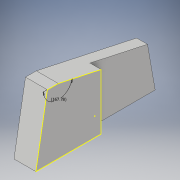
# Autodesk Inventor part: SideProfile
Saved by Autodesk Inventor 2019 (Build 230136000, 136)
## iProperties
Created: 2019-01-04
Part Number: SideProfile
Material: Generic
Document SubType Name: Modeling
Designer: james
Density: 1 g/cm^3
Appearance: Default
Author: james
Autodesk Inventor part; units mm, degrees
ref_plane "YZ Plane" through (0, 0, 0) normal (1, 0, 0) x (0, 1, 0)
ref_plane "XZ Plane" through (0, 0, 0) normal (0, 1, 0) x (-1, 0, 0)
ref_plane "XY Plane" through (0, 0, 0) normal (0, 0, 1) x (1, 0, 0)
sketch "Sketch1" plane through (0, 0, 0) normal (1, 0, 0) x (0, 1, 0)
  line L0 (-43.7628, 137.6658) -> (-43.7628, -167.1342)
  line L1 (-43.7628, -167.1342) -> (57.8372, -149.2194)
  line L2 (-43.7628, 137.6658) -> (108.6372, 110.7936)
  line L3 (108.6372, 110.7936) -> (108.6372, 85.3936)
  line L4 (108.6372, 85.3936) -> (57.8372, -149.2194)
  point P0 (0, 0)
  dimension "d0" = 80
  dimension "d1" = 304.8
  dimension "d2" = 101.6
  dimension "d3" = 80
  dimension "d4" = 152.4
  dimension "d5" = 25.4
  constraints: 10 end point, 2 vertical
  measures "d0" angle of L0 L1
  measures "d1" distance of L0.start L0.end
  measures "d2" distance from line of L0 L1.end
  measures "d3" angle of L2 L0
  measures "d4" distance from line of L0 L2.end
  measures "d5" distance of L2.end L3.end
extrude "Extrusion1" add sketch "Sketch1" along normal blind 25.4
sketch "Sketch2" plane through (25.4, 0, 0) normal (1, 0, 0) x (0, 0, -1)
  line L0 (-137.6658, -43.7628) -> (14.7342, -43.7628)
  line L1 (-137.6658, -43.7628) -> (167.1342, -43.7628) projected
  line L2 (14.7342, -43.7628) -> (14.7342, 86.9569)
  line L3 (149.2194, 57.8372) -> (-85.3936, 108.6372) projected
  line L4 (-85.3936, 108.6372) -> (-110.7936, 108.6372) projected
  line L5 (-110.7936, 108.6372) -> (-137.6658, -43.7628) projected
  point P0 (0, 0)
  dimension "d8" = 152.4
  dimension "d9" = 0
  constraints: 4 end point, 1 midpoint, 1 point on line, 1 vertical
  measures "d8" distance of L0.start L0.end
  measures "d9" distance of L1.start L0.start
extrude "Extrusion2" add sketch "Sketch2" along normal blind 25.4
sketch "Sketch3" plane through (50.8, 0, 0) normal (1, 0, 0) x (0, 0, -1)
  line L0 (-85.3936, 108.6372) -> (-110.7936, 108.6372) projected
  line L1 (-137.6658, -43.7628) -> (14.7342, -43.7628) projected
  line L2 (14.7342, -43.7628) -> (14.7342, 86.9569) projected
  line L3 (14.7342, 86.9569) -> (-85.3936, 108.6372) projected
  line L4 (-85.3936, 108.6372) -> (-110.7936, 108.6372) projected
  line L5 (-110.7936, 108.6372) -> (-137.6658, -43.7628) projected
  point P0 (0, 0)
  dimension "d12" = 167.783
  measures "d12" angle of L0 L3
body "Solid1"
